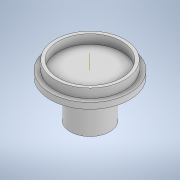
# Autodesk Inventor part: origami_cap
Saved by Autodesk Inventor 2021 (Build 250183000, 183)
## iProperties
Created: 2021-03-04
Part Number: origami_cap
Material: Generic
Document SubType Name: Modeling
Designer: Sihan
Density: 1 g/cm^3
Appearance: Default
Author: Sihan
Autodesk Inventor part; units mm, degrees
ref_plane "YZ Plane" through (0, 0, 0) normal (1, 0, 0) x (0, 1, 0)
ref_plane "XZ Plane" through (0, 0, 0) normal (0, 1, 0) x (-1, 0, 0)
ref_plane "XY Plane" through (0, 0, 0) normal (0, 0, 1) x (1, 0, 0)
sketch "Sketch1" plane through (0, 0, 0) normal (0, 1, 0) x (-1, 0, 0)
  circle A0 centre (0, 0) radius 10
  dimension "d34" = 20
  constraints: 1 centre point
  measures "d34" diameter of A0
extrude "Extrusion1" add sketch "Sketch1" along normal blind 1.5
sketch "Sketch3" plane through (0, 0, 0) normal (1, 0, 0) x (0, 1, 0)
  line L0 (1.5, -8.5901) -> (1.5, 8.5901) projected
  line L1 (1.5, 8.8) -> (3.8, 8.8)
  line L2 (3.8, 8.8) -> (3.8, 8)
  line L3 (3.8, 8) -> (1.5, 8)
  line L4 (-0.8, 0) -> (4.8, 0) projected
  point P0 (0, 0)
  dimension "d3" = 8
  dimension "d4" = 8.8
  dimension "d13" = 2.3
  constraints: 6 end point, 2 point on line, 1 horizontal alignment, 1 parallel, 1 perpendicular
  measures "d3" vertical distance of L2.end point (0, 0)
  measures "d4" vertical distance of point (0, 0) L1.end
  measures "d13" distance between parallel lines of L0 L2
revolve "Revolution1" add sketch "Sketch3" angle 360 about axis through (0, -10, 0) along (0, 1, 0) fills toward (2.65, 8.75) open curves L1 L2 L3
sketch "Sketch7" plane through (0, 0, 0) normal (0, -1, 0) x (1, 0, 0)
  circle A0 centre (0, 0) radius 4.975
  dimension "d35" = 9.95
  constraints: 1 centre point, 1 coincident
  measures "d35" diameter of A0
extrude "Extrusion3" add sketch "Sketch7" along normal blind 1.5
sketch "Sketch8" plane through (0, -1.5, 0) normal (0, -1, 0) x (1, 0, 0)
  circle A0 centre (0, 0) radius 4.975
  constraints: 1 centre point, 1 coincident
extrude "Extrusion4" add sketch "Sketch8" along normal blind 8 separate body
body "Solid1"
body "Solid3"
